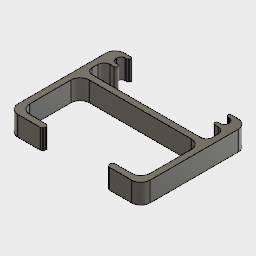
clip main board (Autodesk Fusion 360 design; units mm, degrees)
Autodesk Fusion 360 part; units mm, degrees
sketch "Sketch1" plane through (0, 0, 0) normal (0, 1, 0) x (1, 0, 0)
  line L0 (-12.15, 14.8) -> (-16.65, 14.8)
  line L1 (-16.65, 14.8) -> (-12.15, 14.8)
  line L2 (-12.15, 13.8) -> (-14.15, 13.8)
  line L3 (-15.15, -10.5) -> (-8, -10.5)
  line L4 (-8, -10.5) -> (-8, -12)
  line L5 (-8, -12) -> (-16.65, -12)
  line L6 (-12.15, 13.8) -> (-12.15, 14.8)
  line L7 (-14.15, 13.8) -> (-14.15, 11.5)
  line L8 (-14.15, 11.5) -> (-12.15, 11.5)
  line L9 (-12.15, 11.5) -> (-12.15, 10.5)
  line L10 (-12.15, 10.5) -> (-15.15, 10.5)
  line L11 (-16.65, 14.8) -> (-16.65, -12)
  line L12 (0, 6) -> (-15.15, 6)
  line L13 (-15.15, 6) -> (-15.15, 10.5)
  line L14 (0, 6) -> (0, 4.5)
  line L15 (0, 4.5) -> (-15.15, 4.5)
  line L16 (-15.15, 4.5) -> (-15.15, -10.5)
  dimension "d1" = 2.3
  dimension "d2" = 1
  dimension "d3" = 1
  dimension "d5" = 2
  dimension "d8" = 1.5
  dimension "d11" = 8
  dimension "d13" = 10.5
  dimension "d14" = 10.5
  dimension "d17" = 1
  dimension "d28" = 1.5
  dimension "d29" = 1.5
  dimension "d30" = 4.5
  dimension "d34" = 14.15
  measures "d1" distance of L2.end L7.end
  measures "d2" distance of L8.end L9.end
  measures "d3" distance of L0.start L2.start
  measures "d5" distance of L2.start L2.end
  measures "d8" distance of L3.end L4.end
  measures "d11" distance of origin L4.end
  measures "d13" distance of origin L9.end
  measures "d14" distance of origin L3.end
  measures "d17" distance of L7.end L10.end
  measures "d28" distance of L3.start L5.end
  measures "d29" distance of L12.start L14.end
  measures "d30" distance of L10 L12
  measures "d34" distance of origin L2.end
extrude "Extrude1" add sketch "Sketch1" along normal blind 5 makes body 1
chamfer "Chamfer1" distance 0.5 angle 45 3 edges at (-12.15, 2.5, -13.8) (-8, 2.5, 12) (-8, 2.5, 10.5) on bodies 1
fillet "Fillet1" radius 0.5 6 edges at (-8, 2.5, 11.5) (-8, 2.5, 11) (-8.5, 2.5, 12) (-8.5, 2.5, 10.5) (-12.15, 2.5, -14.3) (-12.65, 2.5, -13.8) on bodies 1
fillet "Fillet2" radius 2.3 4 edges at (-16.65, 2.5, 12) (-16.65, 2.5, -14.8) (-15.15, 2.5, -4.5) (-15.15, 2.5, 10.5) on bodies 1
fillet "Fillet3" radius 0.5 3 edges at (-12.15, 2.5, -14.8) (-12.15, 2.5, -11.5) (-12.15, 2.5, -10.5) on bodies 1
fillet "Fillet4" radius 1 2 edges at (-14.15, 2.5, -13.8) (-14.15, 2.5, -11.5) on bodies 1
fillet "Fillet5" radius 1.5 2 edges at (-15.15, 2.5, -10.5) (-15.15, 2.5, -6) on bodies 1
mirror "Mirror1" about plane through (0, 0, -6) normal (1, 0, 0) of bodies 1 makes body 2
combine "Combine1" operation add target body 1 tool bodies 2
